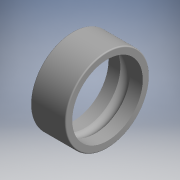
# Autodesk Inventor part: WA673SA Outer ring
Saved by Autodesk Inventor 2017.3 (Build 213256000, 256)
## iProperties
Part Number: WA673SA Outer ring
Material: Generic
Catalog Web Link: www.cadenas.de
Description: Six types or-Metric system sizes
Vendor: NTN
Document SubType Name: Modeling
Designer: partserver
Manufacturer: NTN
Mass: 0.0192773 g
Surface Area: 1.04408 cm^2
Volume: 0.0192773 cm^3
Density: 1 g/cm^3
Appearance: PSOLRGB-192-192-192
Category: PARTsolutions
Company: NTN
Title: WA673SA Outer ring
Author: Cadenas PARTsolutions
Comments: Metric system sizes
PSOL_IDENT_0: {$CADENAS_DATA\23d-libs\ntn\ball_roller_bearings\miniature_extra_small_bb\metric_system_sizes\mss_or
PSOL_IDENT_1: .prj},185 {VTYP=3D},{NB=WA673SA Outer ring},{LINA=WA673SA Outer ring},{NN=Six types or},{DATE=21.12.
PSOL_IDENT_2: 2021 04:23:05},{GEOMDATE=06.03.2020 10:07:12},{VERSION=},{LINEID=11430},{WBVAR=},{WBNUMERIC=}  {NB=W
PSOL_IDENT_3: A673SA Outer ring},{LINA=WA673SA Outer ring},{KT=DUMMY},{IDNR=},{SD=3.0},{D=6},{B=2.0},{R=0.08},{ORD
PSOL_IDENT_4: ER=WA673SA},{CR=242},{COR=94},{CRF=25},{CORF=9,5},{LSG=60 000},{LSO=71 000},{MASS=0.20},{D1=7.2},{D2=
PSOL_IDENT_5: 7.2},{C1=0.6},{C2=0.6},{ORDER1=673},{WSS=WA673SA},{WDS=SSA},{UTWF=FL673},{FORSS=FLWA673SA},{FORDS=SS
PSOL_IDENT_6: A},{DA1=3,6},{DA2=4,1},{DA=5,4},{RAS=0,08},{MASS1=0.26},{B1=2.5},{VERS=2},{X=1.5},{N=9},{O=14.13},{R
PSOL_IDENT_7: B=0.444}
NB: WA673SA Outer ring
NN: Six types or
NT: Metric system sizes
NBSYN: $ORDER. Outer ring
LINA: WA673SA Outer ring
CATALOG: NTN Corporation
SD: 3
D: 6
B: 2
R: 0.08
CR: 242
COR: 94
CRF: 25
CORF: 9,5
LSG: 60 000
LSO: 71 000
MASS: 0.2
D1: 7.2
D2: 7.2
C1: 0.6
C2: 0.6
ORDER1: 673
WSS: WA673SA
WDS: SSA
UTWF: FL673
FORSS: FLWA673SA
FORDS: SSA
DA1: 3,6
DA2: 4,1
DA: 5,4
RAS: 0,08
MASS1: 0.26
B1: 2.5
VERS: 2
SUPPLIER: NTN
ARTICLENO: WA673SA Outer ring
BOMINFO: WA673SA Outer ring
CREATOR: CADENAS GmbH
Autodesk Inventor part; units mm, degrees
sketch "Sketch_2" plane through (0, 0, 0) normal (0, 0, 1) x (1, 0, 0)
  line L0 (2.5, 0) -> (0, 0)
  line L1 (0, 2.92) -> (0, 2.52)
  line L2 (0, 2.52) -> (0.8975, 2.52)
  arc A0 (1.6025, 2.52) -> (0.8975, 2.52) centre (1.25, 2.25) ccw
  line L3 (1.6025, 2.52) -> (2.4438, 2.52)
  line L4 (2.4438, 2.52) -> (2.4438, 2.616)
  line L5 (2.4438, 2.616) -> (2.5, 2.616)
  line L6 (2.5, 2.616) -> (2.5, 2.92)
  arc A1 (2.5, 2.92) -> (2.42, 3) centre (2.42, 2.92) ccw
  line L7 (2.42, 3) -> (0.08, 3)
  arc A2 (0.08, 3) -> (0, 2.92) centre (0.08, 2.92) ccw
  constraints: 16 end point, 6 point on circle, 3 centre point
revolve "Revolution1" add sketch "Sketch_2" angle 360 about axis through (2.5, 0, 0) along (1, 0, 0)
ref_plane "mss_or_XY" through (0, 0, 0) normal (1, 0, 0) x (0, 0, -1)
ref_plane "mss_or_YZ" through (0, 0, 0) normal (0, 0, -1) x (0, 1, 0)
ref_plane "mss_or_ZX" through (0, 0, 0) normal (0, 1, 0) x (1, 0, 0)
ref_plane "mss_or11_XY" through (2.5, 0, 0) normal (1, 0, 0) x (0, 0, -1)
ref_plane "mss_or11_YZ" through (2.5, 0, 0) normal (0, 0, -1) x (0, 1, 0)
ref_plane "mss_or11_ZX" through (2.5, 0, 0) normal (0, 1, 0) x (1, 0, 0)
ref_plane "mss_or2_1_XY" through (1, 2.25, 0) normal (1, 0, 0) x (0, 0, -1)
ref_plane "mss_or2_1_YZ" through (1, 2.25, 0) normal (0, 0, -1) x (0, 1, 0)
ref_plane "mss_or2_1_ZX" through (1, 2.25, 0) normal (0, 1, 0) x (1, 0, 0)
ref_plane "mss_or2_2_XY" through (1, 1.7236, 1.4463) normal (1, 0, 0) x (0, 0, -1)
ref_plane "mss_or2_2_YZ" through (1, 1.7236, 1.4463) normal (0, 0, -1) x (0, 1, 0)
ref_plane "mss_or2_2_ZX" through (1, 1.7236, 1.4463) normal (0, 1, 0) x (1, 0, 0)
ref_plane "mss_or2_3_XY" through (1, 0.3907, 2.2158) normal (1, 0, 0) x (0, 0, -1)
ref_plane "mss_or2_3_YZ" through (1, 0.3907, 2.2158) normal (0, 0, -1) x (0, 1, 0)
ref_plane "mss_or2_3_ZX" through (1, 0.3907, 2.2158) normal (0, 1, 0) x (1, 0, 0)
ref_plane "mss_or2_4_XY" through (1, -1.125, 1.9486) normal (1, 0, 0) x (0, 0, -1)
ref_plane "mss_or2_4_YZ" through (1, -1.125, 1.9486) normal (0, 0, -1) x (0, 1, 0)
ref_plane "mss_or2_4_ZX" through (1, -1.125, 1.9486) normal (0, 1, 0) x (1, 0, 0)
ref_plane "mss_or2_5_XY" through (1, -2.1143, 0.7695) normal (1, 0, 0) x (0, 0, -1)
ref_plane "mss_or2_5_YZ" through (1, -2.1143, 0.7695) normal (0, 0, -1) x (0, 1, 0)
ref_plane "mss_or2_5_ZX" through (1, -2.1143, 0.7695) normal (0, 1, 0) x (1, 0, 0)
ref_plane "mss_or2_6_XY" through (1, -2.1143, -0.7695) normal (1, 0, 0) x (0, 0, -1)
ref_plane "mss_or2_6_YZ" through (1, -2.1143, -0.7695) normal (0, 0, -1) x (0, 1, 0)
ref_plane "mss_or2_6_ZX" through (1, -2.1143, -0.7695) normal (0, 1, 0) x (1, 0, 0)
ref_plane "mss_or2_7_XY" through (1, -1.125, -1.9486) normal (1, 0, 0) x (0, 0, -1)
ref_plane "mss_or2_7_YZ" through (1, -1.125, -1.9486) normal (0, 0, -1) x (0, 1, 0)
ref_plane "mss_or2_7_ZX" through (1, -1.125, -1.9486) normal (0, 1, 0) x (1, 0, 0)
ref_plane "mss_or2_8_XY" through (1, 0.3907, -2.2158) normal (1, 0, 0) x (0, 0, -1)
ref_plane "mss_or2_8_YZ" through (1, 0.3907, -2.2158) normal (0, 0, -1) x (0, 1, 0)
ref_plane "mss_or2_8_ZX" through (1, 0.3907, -2.2158) normal (0, 1, 0) x (1, 0, 0)
ref_plane "mss_or2_9_XY" through (1, 1.7236, -1.4463) normal (1, 0, 0) x (0, 0, -1)
ref_plane "mss_or2_9_YZ" through (1, 1.7236, -1.4463) normal (0, 0, -1) x (0, 1, 0)
ref_plane "mss_or2_9_ZX" through (1, 1.7236, -1.4463) normal (0, 1, 0) x (1, 0, 0)
ref_plane "mss_or21_1_XY" through (1.25, 2.25, 0) normal (1, 0, 0) x (0, 0, -1)
ref_plane "mss_or21_1_YZ" through (1.25, 2.25, 0) normal (0, 0, -1) x (0, 1, 0)
ref_plane "mss_or21_1_ZX" through (1.25, 2.25, 0) normal (0, 1, 0) x (1, 0, 0)
ref_plane "mss_or21_2_XY" through (1.25, 1.7236, 1.4463) normal (1, 0, 0) x (0, 0, -1)
ref_plane "mss_or21_2_YZ" through (1.25, 1.7236, 1.4463) normal (0, 0, -1) x (0, 1, 0)
ref_plane "mss_or21_2_ZX" through (1.25, 1.7236, 1.4463) normal (0, 1, 0) x (1, 0, 0)
ref_plane "mss_or21_3_XY" through (1.25, 0.3907, 2.2158) normal (1, 0, 0) x (0, 0, -1)
ref_plane "mss_or21_3_YZ" through (1.25, 0.3907, 2.2158) normal (0, 0, -1) x (0, 1, 0)
ref_plane "mss_or21_3_ZX" through (1.25, 0.3907, 2.2158) normal (0, 1, 0) x (1, 0, 0)
ref_plane "mss_or21_4_XY" through (1.25, -1.125, 1.9486) normal (1, 0, 0) x (0, 0, -1)
ref_plane "mss_or21_4_YZ" through (1.25, -1.125, 1.9486) normal (0, 0, -1) x (0, 1, 0)
ref_plane "mss_or21_4_ZX" through (1.25, -1.125, 1.9486) normal (0, 1, 0) x (1, 0, 0)
ref_plane "mss_or21_5_XY" through (1.25, -2.1143, 0.7695) normal (1, 0, 0) x (0, 0, -1)
ref_plane "mss_or21_5_YZ" through (1.25, -2.1143, 0.7695) normal (0, 0, -1) x (0, 1, 0)
ref_plane "mss_or21_5_ZX" through (1.25, -2.1143, 0.7695) normal (0, 1, 0) x (1, 0, 0)
ref_plane "mss_or21_6_XY" through (1.25, -2.1143, -0.7695) normal (1, 0, 0) x (0, 0, -1)
ref_plane "mss_or21_6_YZ" through (1.25, -2.1143, -0.7695) normal (0, 0, -1) x (0, 1, 0)
ref_plane "mss_or21_6_ZX" through (1.25, -2.1143, -0.7695) normal (0, 1, 0) x (1, 0, 0)
ref_plane "mss_or21_7_XY" through (1.25, -1.125, -1.9486) normal (1, 0, 0) x (0, 0, -1)
ref_plane "mss_or21_7_YZ" through (1.25, -1.125, -1.9486) normal (0, 0, -1) x (0, 1, 0)
ref_plane "mss_or21_7_ZX" through (1.25, -1.125, -1.9486) normal (0, 1, 0) x (1, 0, 0)
ref_plane "mss_or21_8_XY" through (1.25, 0.3907, -2.2158) normal (1, 0, 0) x (0, 0, -1)
ref_plane "mss_or21_8_YZ" through (1.25, 0.3907, -2.2158) normal (0, 0, -1) x (0, 1, 0)
ref_plane "mss_or21_8_ZX" through (1.25, 0.3907, -2.2158) normal (0, 1, 0) x (1, 0, 0)
ref_plane "mss_or21_9_XY" through (1.25, 1.7236, -1.4463) normal (1, 0, 0) x (0, 0, -1)
ref_plane "mss_or21_9_YZ" through (1.25, 1.7236, -1.4463) normal (0, 0, -1) x (0, 1, 0)
ref_plane "mss_or21_9_ZX" through (1.25, 1.7236, -1.4463) normal (0, 1, 0) x (1, 0, 0)
body "Solid1"
